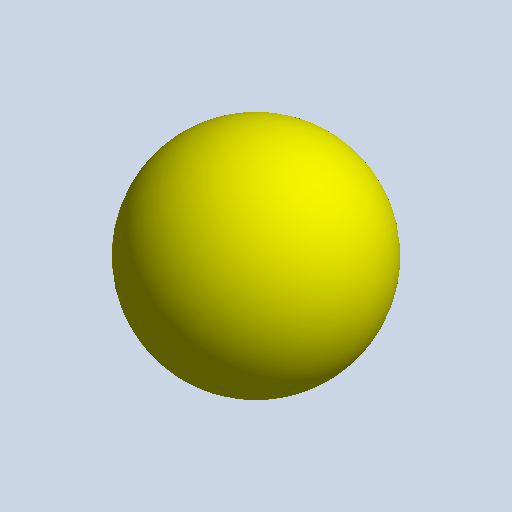
# Autodesk Inventor part: SKF_51102_PART4
Saved by Autodesk Inventor 2022 (Build 260153000, 153)
## iProperties
Part Number: SKF_51102_PART4
Material: Genérico
Catalog Web Link: www.cadenas.de
Description: -Thrust ball bearings, single direction
Vendor: SKF
Document SubType Name: Modeling
Designer: partserver
Manufacturer: SKF
Mass: 23 g
Surface Area: 0.712408 cm^2
Volume: 0.0565414 cm^3
Density: 1 g/cm^3
Appearance: PSOLRGB-192-192-192
Category: PARTsolutions
Company: SKF
PSOL_IDENT_0: {$CADENAS_DATA\23d-libs\skf\bearings_units_and_housings\ball_bearings\thrust_ball_bearings\bd1_001_b
PSOL_IDENT_1: dc_001.prj},207 {VTYP=3D},{NB=SKF_51102_PART4},{LINA=SKF_51102_PART4},{NN=BD1_001_BDC_001_PART4},{NO
PSOL_IDENT_2: PRJ=TRUE},{DATE=21.10.2021 07:35:59},{GEOMDATE=05.07.2021 06:36:39},{VERSION=},{LINEID=46170},{WBVAR=
PSOL_IDENT_3: WASHER},{WBNUMERIC=}  {NB=SKF_51102_PART4},{LINA=SKF_51102_PART4},{KT=DUMMY},{DESIGNATION=51102},{WA
PSOL_IDENT_4: SHER=},{DD=15.0},{D=28.0},{DX=},{DXX=MIN},{H=9.00},{H1=},{DD1=28.00},{D1=16.00},{D2=},{D3=},{C=},{R=
PSOL_IDENT_5: },{SS=},{R12=0.3},{PITCH=21.500},{DW=4.762},{ALPHA=90},{DAMIN=23.00},{DAMAX=20.00},{RAMAX=0.30},{LOA
PSOL_IDENT_6: D1=10.6},{LOAD2=18.3},{LOAD3=0.7},{SPEED1=8500},{SPEED2=12000},{A=0.0017},{Z=12},{II=1},{MASS=0.0230
PSOL_IDENT_7: 0},{BEARING=51102},{WASHERVAR=},{POPULAR=Yes},{XHO=6.4048},{BHO=2.5952},{BSH=2.5952},{Y3=0},{H3=0},{
PSOL_IDENT_8: B3=0},{WASHERALG='','No seat washer'},{WSPN=},{DESIGN=tbb1},{H1ALG=0},{SSALG=0},{RALG=0},{TC=51102},
PSOL_IDENT_9: {DXA=28.000}
NB: SKF_51102_PART4
NT: Thrust ball bearings, single direction
NBSYN: SKF_$TC._PART4
LINA: SKF_51102_PART4
CATALOG: SKF
DESIGNATION: 51102
WASHER: No seat washer
DD: 15
D: 28
H: 9
LOAD1: 10.6
LOAD2: 18.3
LOAD3: 0.7
SPEED1: 8500
SPEED2: 12000
BEARING: 51102
SUPPLIER: SKF
ARTICLENO: SKF_51102_PART4
BOMINFO: SKF_51102_PART4
CREATOR: CADENAS GmbH
Title: SKF_51102_PART4
Author: Cadenas PARTsolutions
Comments: Thrust ball bearings, single direction
Autodesk Inventor part; units mm, degrees
ref_plane "YZ Plane" through (0, 0, 0) normal (1, 0, 0) x (0, 1, 0)
ref_plane "XZ Plane" through (0, 0, 0) normal (0, 1, 0) x (-1, 0, 0)
ref_plane "XY Plane" through (0, 0, 0) normal (0, 0, 1) x (1, 0, 0)
sketch "Sketch_1" plane through (0, 0, 0) normal (0, 0, 1) x (1, 0, 0)
  line L0 (6.881, 10.75) -> (2.119, 10.75)
  arc A0 (6.881, 10.75) -> (2.119, 10.75) centre (4.5, 10.75) ccw
  line L1 (6.881, 10.75) -> (2.119, 10.75)
  dimension "d0" = 360
  constraints: 4 end point, 2 point on circle, 1 centre point
revolve "Revolution1" add sketch "Sketch_1" angle 360 about axis through (6.881, 10.75, 0) along (1, 0, 0)
body "Solid1"
